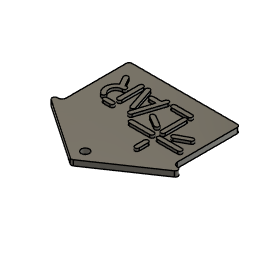
home (Autodesk Fusion 360 design; units mm, degrees)
Autodesk Fusion 360 part; units mm, degrees
sketch "Esboço1" plane through (0, 0, 0) normal (0, 1, 0) x (1, 0, 0)
  line L0 (-19.7256, 15) -> (19.7256, 15)
  line L1 (20.7256, 14) -> (20.7256, -8.5)
  line L2 (-20.7256, -8.5) -> (-20.7256, 14)
  line L3 (22.2256, -10) -> (22.4766, -10)
  line L4 (23.0389, -11.8269) -> (0.5623, -27.111)
  line L5 (-0.5623, -27.111) -> (-23.0389, -11.8269)
  line L6 (-22.4766, -10) -> (-22.2256, -10)
  arc A0 (23.0389, -11.8269) -> (22.4766, -10) centre (22.4766, -11) ccw
  arc A1 (-0.5623, -27.111) -> (0.5623, -27.111) centre (0, -26.2841) ccw
  arc A2 (-22.4766, -10) -> (-23.0389, -11.8269) centre (-22.4766, -11) ccw
  arc A3 (-19.7256, 15) -> (-20.7256, 14) centre (-19.7256, 14) ccw
  arc A4 (20.7256, -8.5) -> (22.2256, -10) centre (22.2256, -8.5) ccw
  arc A5 (-22.2256, -10) -> (-20.7256, -8.5) centre (-22.2256, -8.5) ccw
  arc A6 (20.7256, 14) -> (19.7256, 15) centre (19.7256, 14) ccw
  point P0 (20.7256, -10)
  point P1 (-20.7256, -10)
  point P2 (25.7256, -10)
  point P3 (-25.7256, -10)
  dimension "d25" = 5
  dimension "d26" = 5
  dimension "d29" = 1
  dimension "d30" = 1.5
  dimension "d31" = 1
  constraint horizontal L0
  constraint vertical L1
  constraint vertical L2
  constraint perpendicular L1 L3
  constraint perpendicular L2 L6
  constraint coincident P2 L3
  constraint coincident P2 L4
  constraint tangent L3 A0
  constraint tangent L4 A0
  constraint tangent L4 A1
  constraint tangent L5 A1
  constraint equal A0 A1
  constraint coincident P3 L5
  constraint coincident P3 L6
  constraint tangent L5 A2
  constraint tangent L6 A2
  constraint equal A0 A2
  constraint tangent L0 A3
  constraint tangent L2 A3
  constraint equal A0 A3
  constraint coincident P0 L1
  constraint coincident P0 L3
  constraint tangent L1 A4
  constraint tangent L3 A4
  constraint coincident P1 L2
  constraint coincident P1 L6
  constraint tangent L2 A5
  constraint tangent L6 A5
  constraint equal A4 A5
  constraint tangent L0 A6
  constraint tangent L1 A6
  measures "d25" distance of P0 P2
  measures "d26" distance of P1 P3
  measures "d29" radius of A0
  measures "d30" radius of A4
  measures "d31" radius of A6
extrude "Extrusão1" add sketch "Esboço1" along normal blind 2
sketch "Esboço2" plane through (0, 2, 0) normal (0, 1, 0) x (-1, 0, 0)
  arc A0 (-7.6957, 5.7284) -> (-7.6957, 4.0924) centre (-7.6957, 4.9104) ccw
  arc A1 (9.6001, 3.2824) -> (9.6001, 1.6464) centre (9.6001, 2.4644) ccw
  arc A2 (-8.3998, 11.9964) -> (-10.0358, 11.9964) centre (-9.2178, 11.9964) ccw
  arc A3 (12.1483, 1.6464) -> (12.1483, 3.2824) centre (12.1483, 2.4644) ccw
  arc A4 (-10.5289, 4.1733) -> (-10.5289, 5.8093) centre (-10.5289, 4.9913) ccw
  line L0 (4.3783, -0.0864) -> (7.1036, -8.37) construction
  line L1 (-10.0682, 2.3364) -> (-10.0682, -5.7023)
  line L2 (0.2484, -6.4101) -> (3.8683, -6.4101) construction
  line L3 (-7.6957, 4.9104) -> (-0.0057, 4.9104) construction
  line L4 (-10.0358, 11.9964) -> (-10.0358, 8.5964)
  line L5 (12.4242, -4.9719) -> (14.5369, -8.7718)
  line L6 (9.6001, 1.6464) -> (12.1483, 1.6464)
  line L7 (-8.3998, 8.5964) -> (-8.3998, 11.9964)
  line L8 (-9.2178, 11.9964) -> (-9.2178, 8.5964) construction
  line L9 (-13.1677, 2.533) -> (-17.5076, 0.2031)
  arc A5 (-9.2417, -7.0641) -> (-9.2417, -8.7001) centre (-9.2417, -7.8821) ccw
  line L10 (9.5376, -0.2788) -> (9.5376, -8.3735) construction
  line L11 (-10.5289, 5.8093) -> (-18.2117, 5.8093)
  line L12 (-9.2417, -8.7001) -> (-3.0317, -8.7001)
  arc A6 (-10.0358, 8.5964) -> (-8.3998, 8.5964) centre (-9.2178, 8.5964) ccw
  arc A7 (-12.3938, 1.0916) -> (-13.1677, 2.533) centre (-12.7808, 1.8123) ccw
  line L13 (0.5064, -8.266) -> (3.7944, 1.8702)
  line L14 (-7.6957, 4.0924) -> (-0.0057, 4.0924)
  line L15 (-0.0057, 5.7284) -> (-7.6957, 5.7284)
  arc A8 (-8.4322, 2.3364) -> (-10.0682, 2.3364) centre (-9.2502, 2.3364) ccw
  arc A9 (-0.0057, 4.0924) -> (-0.0057, 5.7284) centre (-0.0057, 4.9104) ccw
  arc A10 (3.7944, 1.8702) -> (2.2383, 2.375) centre (3.0163, 2.1226) ccw
  line L16 (12.1483, 3.2824) -> (9.6001, 3.2824)
  line L17 (0.2484, -7.2281) -> (3.8683, -7.2281)
  line L18 (-16.7338, -1.2383) -> (-12.3938, 1.0916)
  arc A11 (12.141, -4.7193) -> (14.2741, 0.968) centre (12.1819, -1.4909) ccw construction
  arc A12 (13.854, -4.1769) -> (12.4242, -4.9719) centre (13.1391, -4.5744) ccw
  arc A13 (14.5369, -8.7718) -> (15.9667, -7.9767) centre (15.2518, -8.3742) ccw
  line L19 (2.2383, 2.375) -> (-1.0498, -7.7612)
  arc A14 (5.1554, 0.1693) -> (3.6013, -0.342) centre (4.3783, -0.0864) ccw
  line L20 (9.6001, 2.4644) -> (12.1483, 2.4644) construction
  arc A15 (-17.5076, 0.2031) -> (-16.7338, -1.2383) centre (-17.1207, -0.5176) ccw
  line L21 (8.7196, -0.2788) -> (8.7196, -8.3735)
  line L22 (3.6013, -0.342) -> (6.3265, -8.6256)
  arc A16 (12.1514, -3.9012) -> (12.1306, -5.5373) centre (12.141, -4.7193) ccw
  arc A17 (12.1514, -3.9012) -> (13.7439, 0.3449) centre (12.1819, -1.4909) ccw
  arc A18 (-1.0498, -7.7612) -> (0.5064, -8.266) centre (-0.2717, -8.0136) ccw
  arc A19 (6.3265, -8.6256) -> (7.8806, -8.1144) centre (7.1036, -8.37) ccw
  arc A20 (3.8683, -7.2281) -> (3.8683, -5.5921) centre (3.8683, -6.4101) ccw
  line L23 (13.1391, -4.5744) -> (15.2518, -8.3742) construction
  arc A21 (12.1306, -5.5373) -> (14.8043, 1.5911) centre (12.1819, -1.4909) ccw
  line L24 (-6.0435, 1.3999) -> (-2.2156, -0.8491) construction
  line L25 (-6.4578, 0.6946) -> (-2.63, -1.5544)
  arc A22 (-3.0317, -8.7001) -> (-3.0317, -7.0641) centre (-3.0317, -7.8821) ccw
  arc A23 (10.3556, -0.2788) -> (8.7196, -0.2788) centre (9.5376, -0.2788) ccw
  line L26 (10.3556, -8.3735) -> (10.3556, -0.2788)
  line L27 (7.8806, -8.1144) -> (5.1554, 0.1693)
  line L28 (-1.8012, -0.1438) -> (-5.6291, 2.1051)
  arc A24 (0.2484, -5.5921) -> (0.2484, -7.2281) centre (0.2484, -6.4101) ccw
  line L29 (3.8683, -5.5921) -> (0.2484, -5.5921)
  arc A25 (-5.6291, 2.1051) -> (-6.4578, 0.6946) centre (-6.0435, 1.3999) ccw
  arc A26 (-2.63, -1.5544) -> (-1.8012, -0.1438) centre (-2.2156, -0.8491) ccw
  arc A27 (8.7196, -8.3735) -> (10.3556, -8.3735) centre (9.5376, -8.3735) ccw
  line L30 (-3.0317, -7.0641) -> (-9.2417, -7.0641)
  line L31 (-10.5289, 4.9913) -> (-18.2117, 4.9913) construction
  line L32 (-8.4322, -5.7023) -> (-8.4322, 2.3364)
  line L33 (-9.2417, -7.8821) -> (-3.0317, -7.8821) construction
  line L34 (-18.2117, 4.1733) -> (-10.5289, 4.1733)
  line L35 (15.9667, -7.9767) -> (13.854, -4.1769)
  line L36 (-17.1207, -0.5176) -> (-12.7808, 1.8123) construction
  arc A28 (-18.2117, 5.8093) -> (-18.2117, 4.1733) centre (-18.2117, 4.9913) ccw
  arc A29 (14.8043, 1.5911) -> (13.7439, 0.3449) centre (14.2741, 0.968) ccw
  line L37 (-0.2717, -8.0136) -> (3.0163, 2.1226) construction
  line L38 (-9.2502, 2.3364) -> (-9.2502, -5.7023) construction
  arc A30 (-10.0682, -5.7023) -> (-8.4322, -5.7023) centre (-9.2502, -5.7023) ccw
  line L39 (23.0389, 11.8269) -> (0.5623, 27.111)
  line L40 (-0.5623, 27.111) -> (-23.0389, 11.8269)
  line L41 (-22.4766, 10) -> (-22.2256, 10)
  line L42 (-20.7256, 8.5) -> (-20.7256, -14)
  line L43 (-19.7256, -15) -> (19.7256, -15)
  line L44 (20.7256, -14) -> (20.7256, 8.5)
  line L45 (22.2256, 10) -> (22.4766, 10)
  arc A31 (19.7256, -15) -> (20.7256, -14) centre (19.7256, -14) ccw
  arc A32 (22.4766, 10) -> (23.0389, 11.8269) centre (22.4766, 11) ccw
  arc A33 (0.5623, 27.111) -> (-0.5623, 27.111) centre (0, 26.2841) ccw
  arc A34 (-23.0389, 11.8269) -> (-22.4766, 10) centre (-22.4766, 11) ccw
  arc A35 (-20.7256, 8.5) -> (-22.2256, 10) centre (-22.2256, 8.5) ccw
  arc A36 (22.2256, 10) -> (20.7256, 8.5) centre (22.2256, 8.5) ccw
  arc A37 (-20.7256, -14) -> (-19.7256, -15) centre (-19.7256, -14) ccw
  point P0 (-1.3, 2)
  point P1 (-1.3, 2)
  point P2 (2.75, -13.35)
  point P3 (2.75, -13.35)
  point P4 (3.3879, -13.4686)
  point P5 (2.75, -13.35)
  point P6 (2.75, -13.35)
  point P7 (2.75, -13.35)
  dimension "d4" = 1.6362
  dimension "d5" = 1.636
  dimension "d6" = 1.636
  dimension "d7" = 1.636
  dimension "d8" = 1.636
  dimension "d9" = 1.636
  dimension "d10" = 1.636
  dimension "d11" = 1.636
  dimension "d12" = 1.636
  dimension "d13" = 4.4396
  dimension "d14" = 1.636
  dimension "d15" = 1.636
  dimension "d16" = 1.636
  dimension "d17" = 1.636
  dimension "d18" = 1.636
  dimension "d19" = 3.4
  constraint coincident P0 P1
  constraint tangent L4 A6
  constraint tangent L7 A6
  constraint parallel L4 L7
  constraint tangent A2 L7
  constraint tangent A2 L4
  constraint tangent L14 A9
  constraint tangent L15 A9
  constraint parallel L14 L15
  constraint tangent A0 L15
  constraint tangent A0 L14
  constraint tangent L25 A26
  constraint tangent L28 A26
  constraint parallel L25 L28
  constraint tangent L28 A25
  constraint tangent L25 A25
  constraint tangent L1 A30
  constraint tangent L32 A30
  constraint parallel L1 L32
  constraint tangent A8 L32
  constraint tangent L1 A8
  constraint tangent A7 L18
  constraint tangent L9 A7
  constraint parallel L9 L18
  constraint tangent L9 A15
  constraint tangent L18 A15
  constraint tangent L11 A28
  constraint tangent L34 A28
  constraint parallel L11 L34
  constraint tangent A4 L34
  constraint tangent A4 L11
  constraint perpendicular L1 L31
  constraint tangent L12 A22
  constraint tangent A22 L30
  constraint parallel L12 L30
  constraint tangent A5 L30
  constraint tangent A5 L12
  constraint perpendicular L1 L33
  constraint tangent L13 A10
  constraint tangent A10 L19
  constraint parallel L13 L19
  constraint tangent L19 A18
  constraint tangent L13 A18
  constraint tangent L17 A20
  constraint tangent A20 L29
  constraint parallel L17 L29
  constraint tangent A24 L29
  constraint tangent L17 A24
  constraint coincident L2.start L37
  constraint tangent L22 A19
  constraint tangent A19 L27
  constraint parallel L22 L27
  constraint tangent A14 L27
  constraint tangent A14 L22
  constraint tangent L21 A27
  constraint tangent L26 A27
  constraint parallel L21 L26
  constraint tangent A23 L26
  constraint tangent L21 A23
  constraint tangent A3 L6
  constraint tangent A3 L16
  constraint parallel L6 L16
  constraint tangent A1 L16
  constraint tangent A1 L6
  constraint tangent A16 A21
  constraint tangent A16 A17
  constraint tangent A17 A29
  constraint tangent A21 A29
  constraint tangent L5 A13
  constraint tangent A13 L35
  constraint parallel L5 L35
  constraint tangent A12 L35
  constraint tangent L5 A12
  constraint coincident A12.centre A11
  measures "d4" distance of A17 A21
  measures "d5" distance of L6 L16
  measures "d6" distance of L5 L35
  measures "d7" distance of L21 L26
  measures "d8" distance of L22 L27
  measures "d9" distance of L17 L29
  measures "d10" distance of L13 L19
  measures "d11" distance of L12 L30
  measures "d12" distance of L1 L32
  measures "d13" distance of L24.end L24.start
  measures "d14" distance of L25 L28
  measures "d15" distance of L14 L15
  measures "d16" distance of L11 L34
  measures "d17" distance of L4 L7
  measures "d18" distance of L9 L18
  measures "d19" distance of A2.centre L8.end
extrude "Extrusão2" add sketch "Esboço2" along normal blind 1 contours A0 L14 L15 A9 | A1 A3 L6 L16 | A2 L4 L7 A6 | A4 L11 L34 A28 | L1 A8 L32 A30 | L5 A12 A21 L35 | L5 A12 A16 A17 A21 | L5 A13 A21 L35 | A12 A17 A21 L35 A29 | L9 A7 L18 A15 | A5 L12 A22 L30 | L13 L17 L19 A18 A24 | L13 L17 A24 L29 | L13 L17 A20 L29 | L13 A10 L19 A24 L29 | A14 L22 A19 L27 | L21 A23 L26 A27 | L25 L28 A25 A26
sketch "Esboço3" plane through (0, 2, 0) normal (0, 1, 0) x (-1, 0, 0)
  arc A0 (12.1483, 1.6464) -> (12.1483, 3.2824) centre (12.1483, 2.4644) ccw
  line L0 (12.1483, 1.6464) -> (9.6001, 1.6464)
  arc A1 (9.6001, 3.2824) -> (9.6001, 1.6464) centre (9.6001, 2.4644) ccw
  line L1 (9.6001, 3.2824) -> (12.1483, 3.2824)
  arc A2 (3.8683, -7.2281) -> (3.8683, -5.5921) centre (3.8683, -6.4101) ccw
  line L2 (3.8683, -7.2281) -> (0.843, -7.2281)
  line L3 (0.843, -7.2281) -> (0.5064, -8.266)
  arc A3 (-1.0498, -7.7612) -> (0.5064, -8.266) centre (-0.2717, -8.0136) ccw
  line L4 (-1.0498, -7.7612) -> (2.2383, 2.375)
  arc A4 (3.7944, 1.8702) -> (2.2383, 2.375) centre (3.0163, 2.1226) ccw
  line L5 (3.7944, 1.8702) -> (1.3737, -5.5921)
  line L6 (1.3737, -5.5921) -> (3.8683, -5.5921)
  line L7 (-10.0682, -5.7023) -> (-10.0682, 2.3364)
  arc A5 (-8.4322, 2.3364) -> (-10.0682, 2.3364) centre (-9.2502, 2.3364) ccw
  line L8 (-8.4322, 2.3364) -> (-8.4322, -5.7023)
  arc A6 (-10.0682, -5.7023) -> (-8.4322, -5.7023) centre (-9.2502, -5.7023) ccw
  line L9 (-10.0358, 8.5964) -> (-10.0358, 11.9964)
  arc A7 (-8.3998, 11.9964) -> (-10.0358, 11.9964) centre (-9.2178, 11.9964) ccw
  line L10 (-8.3998, 11.9964) -> (-8.3998, 8.5964)
  arc A8 (-10.0358, 8.5964) -> (-8.3998, 8.5964) centre (-9.2178, 8.5964) ccw
  line L11 (-2.63, -1.5544) -> (-6.4578, 0.6946)
  arc A9 (-5.6291, 2.1051) -> (-6.4578, 0.6946) centre (-6.0435, 1.3999) ccw
  line L12 (-5.6291, 2.1051) -> (-1.8012, -0.1438)
  arc A10 (-2.63, -1.5544) -> (-1.8012, -0.1438) centre (-2.2156, -0.8491) ccw
  arc A11 (6.3265, -8.6256) -> (7.8806, -8.1144) centre (7.1036, -8.37) ccw
  line L13 (6.3265, -8.6256) -> (3.6013, -0.342)
  arc A12 (5.1554, 0.1693) -> (3.6013, -0.342) centre (4.3783, -0.0864) ccw
  line L14 (5.1554, 0.1693) -> (7.8806, -8.1144)
  arc A13 (12.1514, -3.9012) -> (13.7439, 0.3449) centre (12.1819, -1.4909) ccw
  arc A14 (14.8043, 1.5911) -> (13.7439, 0.3449) centre (14.2741, 0.968) ccw
  arc A15 (14.2834, -4.9492) -> (14.8043, 1.5911) centre (12.1819, -1.4909) ccw
  line L15 (14.2834, -4.9492) -> (15.9667, -7.9767)
  arc A16 (14.5369, -8.7718) -> (15.9667, -7.9767) centre (15.2518, -8.3742) ccw
  line L16 (14.5369, -8.7718) -> (12.7188, -5.5019)
  arc A17 (12.1306, -5.5373) -> (12.7188, -5.5019) centre (12.1819, -1.4909) ccw
  arc A18 (12.1514, -3.9012) -> (12.1306, -5.5373) centre (12.141, -4.7193) ccw
  arc A19 (-3.0317, -8.7001) -> (-3.0317, -7.0641) centre (-3.0317, -7.8821) ccw
  line L17 (-3.0317, -8.7001) -> (-9.2417, -8.7001)
  arc A20 (-9.2417, -7.0641) -> (-9.2417, -8.7001) centre (-9.2417, -7.8821) ccw
  line L18 (-9.2417, -7.0641) -> (-3.0317, -7.0641)
  line L19 (-17.5076, 0.2031) -> (-13.1677, 2.533)
  arc A21 (-12.3938, 1.0916) -> (-13.1677, 2.533) centre (-12.7808, 1.8123) ccw
  line L20 (-12.3938, 1.0916) -> (-16.7338, -1.2383)
  arc A22 (-17.5076, 0.2031) -> (-16.7338, -1.2383) centre (-17.1207, -0.5176) ccw
  line L21 (-18.2117, 5.8093) -> (-10.5289, 5.8093)
  arc A23 (-10.5289, 4.1733) -> (-10.5289, 5.8093) centre (-10.5289, 4.9913) ccw
  line L22 (-10.5289, 4.1733) -> (-18.2117, 4.1733)
  arc A24 (-18.2117, 5.8093) -> (-18.2117, 4.1733) centre (-18.2117, 4.9913) ccw
  line L23 (-0.0057, 4.0924) -> (-7.6957, 4.0924)
  arc A25 (-7.6957, 5.7284) -> (-7.6957, 4.0924) centre (-7.6957, 4.9104) ccw
  line L24 (-7.6957, 5.7284) -> (-0.0057, 5.7284)
  arc A26 (-0.0057, 4.0924) -> (-0.0057, 5.7284) centre (-0.0057, 4.9104) ccw
  line L25 (8.7196, -8.3735) -> (8.7196, -0.2788)
  arc A27 (10.3556, -0.2788) -> (8.7196, -0.2788) centre (9.5376, -0.2788) ccw
  line L26 (10.3556, -0.2788) -> (10.3556, -8.3735)
  arc A28 (8.7196, -8.3735) -> (10.3556, -8.3735) centre (9.5376, -8.3735) ccw
  circle A29 centre (-0.0421, 22.1477) radius 1.5
  line L27 (23.0389, 11.8269) -> (0.5623, 27.111)
  line L28 (-0.5623, 27.111) -> (-23.0389, 11.8269)
  line L29 (-22.4766, 10) -> (-22.2256, 10)
  line L30 (-20.7256, 8.5) -> (-20.7256, -14)
  line L31 (-19.7256, -15) -> (19.7256, -15)
  line L32 (20.7256, -14) -> (20.7256, 8.5)
  line L33 (22.2256, 10) -> (22.4766, 10)
  arc A30 (19.7256, -15) -> (20.7256, -14) centre (19.7256, -14) ccw
  arc A31 (22.4766, 10) -> (23.0389, 11.8269) centre (22.4766, 11) ccw
  arc A32 (0.5623, 27.111) -> (-0.5623, 27.111) centre (0, 26.2841) ccw
  arc A33 (-23.0389, 11.8269) -> (-22.4766, 10) centre (-22.4766, 11) ccw
  arc A34 (-20.7256, 8.5) -> (-22.2256, 10) centre (-22.2256, 8.5) ccw
  arc A35 (22.2256, 10) -> (20.7256, 8.5) centre (22.2256, 8.5) ccw
  arc A36 (-20.7256, -14) -> (-19.7256, -15) centre (-19.7256, -14) ccw
  dimension "d22" = 3
  dimension "d28" = 5
  measures "d22" diameter of A29
  measures "d28" distance of A29.centre L27.end
extrude "Extrusão3" cut sketch "Esboço3" against normal blind 6 contours A29
